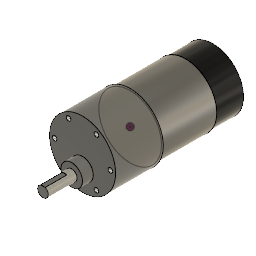
Motor Mount v8 (Autodesk Fusion 360 archive; units mm, degrees)
design "37D 131-1 Gearbox Motor"
Autodesk Fusion 360 part; units mm, degrees
note: some values were not read from the file. Chosen so that the rebuilt part matches the saved one: which face or edge a step refers to; how an offset face is resized. Set by a fixed rule: which sketch regions a step uses.
sketch "Skizze1" plane through (0, 0, 0) normal (0, 1, 0) x (1, 0, 0)
  circle A0 centre (0, 0) radius 17.4
  dimension "d1" = 34.8
  dimension "d62" = 0
  dimension "d63" = 0
  dimension "d64" = 0
  dimension "d65" = 0
  dimension "d74" = 0
  dimension "d75" = 0
  dimension "d76" = 0
  dimension "d77" = 0
  dimension "d86" = 0
  dimension "d87" = 0
  dimension "d88" = 0
  dimension "d89" = 0
  measures "d1" diameter of A0
extrude "Extrusion3" add sketch "Skizze1" along normal blind 30.7 makes body 1
extrude "Extrusion2" add sketch "Skizze1" along normal blind 30.7 separate body makes body 2
extrude "Extrusion1" add sketch "Skizze1" along normal blind 30.7 separate body makes body 3
copy_body "Körper->Berechn1" bodies 1 removing the originals makes body 4 in component "Motor"
ref_plane "Arbeitsebene1" through (0, 0, 0) normal (0, 1, 0) x (1, 0, 0) in component "Gearbox"
sketch "Skizze1 (2)" plane through (0, 0, 0) normal (0, 1, 0) x (1, 0, 0) in component "Gearbox"
  circle A0 centre (0, 0) radius 18.4
  dimension "d13" = 36.8
  measures "d13" diameter of A0
extrude "Extrusion1'" add sketch "Skizze1 (2)" against normal blind 26.5 separate body makes body 5 in component "Gearbox"
ref_plane "Arbeitsebene1" through (0, 30.7, 0) normal (0, 1, 0) x (1, 0, 0) in component "Encoder"
sketch "Skizze1 (3)" plane through (0, 30.7, 0) normal (0, 1, 0) x (1, 0, 0) in component "Encoder"
  circle A0 centre (0, 0) radius 17
  dimension "d17" = 34
  measures "d17" diameter of A0
extrude "Extrusion1''" add sketch "Skizze1 (3)" along normal blind 15.4 separate body makes body 6 in component "Encoder"
sketch "Skizze3" plane through (0, -26.5, 0) normal (0, -1, 0) x (1, 0, 0)
  circle A0 centre (0, 0) radius 18.4
  circle A1 centre (0, 0) radius 15.5 construction
  circle A2 centre (0, -7) radius 6
  line L0 (0, 0) -> (0, -28) construction
  dimension "d20" = 31
  dimension "d21" = 12
  dimension "d22" = 7
  measures "d20" diameter of A1
  measures "d21" diameter of A2
  measures "d22" distance of A0.centre
extrude "Extrusion2'" add sketch "Skizze3" along normal blind 6 contours A2 bodies 5 in component "Gearbox"
sketch "Skizze4" plane through (0, -32.5, 0) normal (0, -1, 0) x (1, 0, 0)
  circle A0 centre (0, -7) radius 6
  circle A1 centre (0, -7) radius 3
  dimension "d25" = 6
  measures "d25" diameter of A1
extrude "Extrusion3'" add sketch "Skizze4" along normal blind 16 contours A1 bodies 5 in component "Gearbox"
sketch "Skizze2" plane through (0, -26.5, 0) normal (0, -1, 0) x (1, 0, 0) in component "Gearbox"
  circle A0 centre (0, -7) radius 6
  circle A1 centre (0, 0) radius 18.4
  circle A2 centre (0, 0) radius 15.5 construction
  circle A3 centre (-15.5, 0) radius 1.6
  circle A4 centre (-7.75, -13.4234) radius 1.6
  circle A5 centre (7.75, -13.4234) radius 1.6
  circle A6 centre (15.5, 0) radius 1.6
  circle A7 centre (7.75, 13.4234) radius 1.6
  circle A8 centre (-7.75, 13.4234) radius 1.6
  dimension "d28" = 31
  dimension "d29" = 3.2
  dimension "d31" = 360
  measures "d28" diameter of A2
  measures "d29" diameter of A3
extrude "Extrusion4" cut sketch "Skizze2" against normal blind 3 contours A3 | A4 | A5 | A6 | A7 | A8 bodies 5 in component "Gearbox"
thread "Gewinde1" "ISO Metric profile 3.0 M3x0.5 6H" major diameter 3.086 minor diameter 2.529 pitch 0.5 angle 60 resizes the face on face at (-6.152, -24.5, 13.3436) on bodies 5 in component "Gearbox"
thread "Gewinde2" "ISO Metric profile 3.0 M3x0.5 6H" major diameter 3.086 minor diameter 2.529 pitch 0.5 angle 60 resizes the face on face at (9.348, -24.5, 13.3436) on bodies 5 in component "Gearbox"
thread "Gewinde3" "ISO Metric profile 3.0 M3x0.5 6H" major diameter 3.086 minor diameter 2.529 pitch 0.5 angle 60 resizes the face on face at (17.098, -24.5, -0.0798) on bodies 5 in component "Gearbox"
thread "Gewinde4" "ISO Metric profile 3.0 M3x0.5 6H" major diameter 3.086 minor diameter 2.529 pitch 0.5 angle 60 resizes the face on face at (-13.902, -24.5, -0.0798) on bodies 5 in component "Gearbox"
thread "Gewinde5" "ISO Metric profile 3.0 M3x0.5 6H" major diameter 3.086 minor diameter 2.529 pitch 0.5 angle 60 resizes the face on face at (-6.152, -24.5, -13.5031) on bodies 5 in component "Gearbox"
thread "Gewinde6" "ISO Metric profile 3.0 M3x0.5 6H" major diameter 3.086 minor diameter 2.529 pitch 0.5 angle 60 resizes the face on face at (9.348, -24.5, -13.5031) on bodies 5 in component "Gearbox"
sketch "Skizze5" plane through (0, -48.5, 0) normal (0, -1, 0) x (1, 0, 0)
  circle A0 centre (0, -7) radius 3
  line L0 (-3, -2.3) -> (3, -2.3)
  line L1 (3, -2.3) -> (3, -4.3)
  line L2 (3, -4.3) -> (-3, -4.3)
  line L3 (-3, -4.3) -> (-3, -2.3)
  dimension "d130" = 2.7
extrude "Extrusion5" cut sketch "Skizze5" against normal blind 12 contours A0 L2 | A0 L0 L1 L2 L3 picked at (-0.0644, -4.105) bodies 5 in component "Gearbox"
component "Motor" placed x (1, 0, 0) y (0, 1, 0) z (0, 0, 1) at (0, 0, 0)
component "Gearbox" placed x (1, 0, 0) y (0, 1, 0) z (0, 0, 1) at (0, 0, 0)
component "Encoder" placed x (1, 0, 0) y (0, 1, 0) z (0, 0, 1) at (0, 0, 0)
